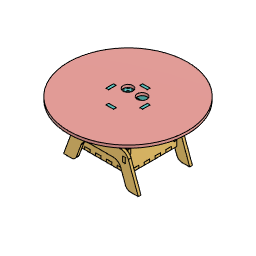
finalprojectbuild (Autodesk Fusion 360 design; units mm, degrees)
Autodesk Fusion 360 part; units mm, degrees
(part 1 of 2)
sketch "Sketch1" plane through (0, 0, 0) normal (1, 0, 0) x (0, 1, 0)
  line L0 (45, 50) -> (40, 50)
  line L1 (50, 45) -> (55, 45)
  line L2 (65, 50) -> (60, 50)
  line L3 (35, 45) -> (30, 45)
  line L4 (20, 50) -> (25, 50)
  line L5 (15, 45) -> (10, 45)
  line L6 (70, 45) -> (75, 45)
  line L7 (45, 50) -> (40, 50)
  line L8 (65, 50) -> (60, 50)
  line L9 (0, 50) -> (5, 50)
  line L10 (20, 50) -> (25, 50)
  line L11 (25, 50) -> (20, 50)
  line L12 (5, 50) -> (0, 50)
  line L13 (45, 0) -> (40, 0)
  line L14 (65, 0) -> (60, 0)
  line L15 (65, 0) -> (60, 0)
  line L16 (20, 0) -> (25, 0)
  line L17 (45, 0) -> (40, 0)
  line L18 (20, 0) -> (25, 0)
  line L19 (25, 0) -> (20, 0)
  line L20 (0, 0) -> (5, 0)
  line L21 (20, 0) -> (25, 0)
  line L22 (40, 0) -> (45, 0)
  line L23 (60, 0) -> (65, 0)
  line L24 (5, 30) -> (0, 30)
  line L25 (0, 20) -> (5, 20)
  line L26 (5, 20) -> (0, 20)
  line L27 (0, 10) -> (5, 10)
  line L28 (5, 10) -> (5, 20)
  line L29 (5, 30) -> (0, 30)
  line L30 (0, 40) -> (5, 40)
  line L31 (5, 40) -> (5, 30)
  line L32 (0, 20) -> (-5, 20)
  line L33 (-5, 20) -> (-5, 30)
  line L34 (-5, 30) -> (0, 30)
  line L35 (0, 50) -> (0, 40)
  line L36 (0, 10) -> (0, 0)
  line L37 (0, 50) -> (0, 40)
  line L38 (80, 45) -> (80, 50)
  line L39 (5, 50) -> (10, 50)
  line L40 (10, 50) -> (10, 45)
  line L41 (20, 50) -> (20, 45)
  line L42 (20, 45) -> (10, 45)
  line L43 (10, 45) -> (10, 50)
  line L44 (30, 45) -> (30, 50)
  line L45 (30, 50) -> (20, 50)
  line L46 (20, 50) -> (20, 45)
  line L47 (40, 50) -> (40, 45)
  line L48 (40, 45) -> (30, 45)
  line L49 (30, 45) -> (30, 50)
  line L50 (50, 45) -> (50, 50)
  line L51 (50, 50) -> (40, 50)
  line L52 (40, 50) -> (40, 45)
  line L53 (50, 45) -> (60, 45)
  line L54 (60, 45) -> (60, 50)
  line L55 (50, 50) -> (50, 45)
  line L56 (70, 45) -> (70, 50)
  line L57 (70, 50) -> (60, 50)
  line L58 (60, 50) -> (60, 45)
  line L59 (70, 45) -> (80, 45)
  line L60 (80, 45) -> (80, 50)
  line L61 (70, 50) -> (70, 45)
  line L62 (90, 45) -> (90, 50)
  line L63 (90, 50) -> (80, 50)
  line L64 (80, 50) -> (80, 45)
  line L65 (80, 45) -> (75, 45)
  line L66 (80, 0) -> (90, 0)
  line L67 (85, 40) -> (85, 30)
  line L68 (90, 10) -> (85, 10)
  line L69 (85, 30) -> (90, 30)
  line L70 (85, 30) -> (90, 30)
  line L71 (85, 20) -> (90, 20)
  line L72 (95, 20) -> (95, 30)
  line L73 (95, 30) -> (90, 30)
  line L74 (85, 10) -> (85, 20)
  line L75 (90, 20) -> (95, 20)
  line L76 (90, 40) -> (85, 40)
  line L77 (90, 20) -> (85, 20)
  line L78 (90, 40) -> (90, 45)
  line L79 (90, 0) -> (90, 10)
  line L80 (90, 50) -> (90, 25)
  line L81 (90, 25) -> (58, 25)
  line L82 (40, 5) -> (30, 5)
  line L83 (20, 0) -> (25, 0)
  line L84 (40, 0) -> (40, 5)
  line L85 (30, 5) -> (30, 0)
  line L86 (50, 5) -> (55, 5)
  line L87 (70, 5) -> (75, 5)
  line L88 (35, 5) -> (30, 5)
  line L89 (15, 5) -> (10, 5)
  line L90 (70, 0) -> (60, 0)
  line L91 (45, 0) -> (40, 0)
  line L92 (30, 0) -> (20, 0)
  line L93 (10, 0) -> (10, 5)
  line L94 (80, 5) -> (80, 0)
  line L95 (50, 5) -> (60, 5)
  line L96 (40, 0) -> (40, 5)
  line L97 (65, 0) -> (60, 0)
  line L98 (10, 5) -> (10, 0)
  line L99 (50, 0) -> (40, 0)
  line L100 (70, 0) -> (70, 5)
  line L101 (80, 5) -> (75, 5)
  line L102 (70, 5) -> (80, 5)
  line L103 (20, 0) -> (25, 0)
  line L104 (45, 0) -> (40, 0)
  line L105 (80, 5) -> (80, 0)
  line L106 (20, 0) -> (20, 5)
  line L107 (70, 5) -> (70, 0)
  line L108 (60, 0) -> (60, 5)
  line L109 (65, 0) -> (60, 0)
  line L110 (80, 0) -> (80, 5)
  line L111 (20, 0) -> (20, 5)
  line L112 (20, 5) -> (10, 5)
  line L113 (50, 0) -> (50, 5)
  line L114 (30, 5) -> (30, 0)
  line L115 (25, 0) -> (20, 0)
  line L116 (60, 5) -> (60, 0)
  line L117 (50, 5) -> (50, 0)
  line L118 (5, 0) -> (10, 0)
  line L119 (20, 0) -> (30, 0)
  line L120 (40, 0) -> (50, 0)
  line L121 (60, 0) -> (70, 0)
  line L122 (80, 0) -> (90, 0)
  dimension "d1" = 80
  dimension "d2" = 50
  dimension "d3" = 40
  dimension "d19" = 5
  dimension "d20" = 10
  dimension "d21" = 5
  dimension "d22" = 10
  dimension "d23" = 5
  dimension "d24" = 10
  dimension "d55" = 5
  dimension "d57" = 10
  dimension "d58" = 5
  dimension "d59" = 10
  dimension "d60" = 5
  dimension "d61" = 10
  dimension "d62" = 5
  dimension "d63" = 10
  dimension "d64" = 10
  dimension "d65" = 10
  dimension "d66" = 10
  dimension "d67" = 10
  dimension "d73" = 85
  dimension "d74" = 25
  dimension "d75" = 32
  constraint horizontal L20
  constraint vertical L35
  constraint coincident L20.start L36.end
  constraint perpendicular L9 L35
  constraint horizontal L0
  constraint horizontal L1
  constraint horizontal L2
  constraint horizontal L3
  constraint horizontal L4
  constraint horizontal L5
  constraint horizontal L6
  constraint collinear L9 L10
  constraint collinear L11 L12
  constraint perpendicular L5 L37
  constraint collinear L20 L21
  constraint collinear L21 L22
  constraint collinear L22 L23
  constraint horizontal L24
  constraint horizontal L25
  constraint horizontal L26
  constraint horizontal L27
  constraint vertical L28
  constraint horizontal L29
  constraint horizontal L30
  constraint vertical L31
  constraint horizontal L32
  constraint vertical L33
  constraint horizontal L34
  constraint collinear L35 L36
  constraint horizontal L39
  constraint vertical L40
  constraint vertical L41
  constraint horizontal L42
  constraint vertical L43
  constraint vertical L44
  constraint horizontal L45
  constraint vertical L46
  constraint vertical L47
  constraint horizontal L48
  constraint vertical L49
  constraint vertical L50
  constraint horizontal L51
  constraint vertical L52
  constraint horizontal L53
  constraint vertical L54
  constraint vertical L55
  constraint vertical L56
  constraint horizontal L57
  constraint vertical L58
  constraint horizontal L59
  constraint vertical L60
  constraint vertical L61
  constraint vertical L62
  constraint horizontal L63
  constraint vertical L64
  constraint horizontal L65
  constraint horizontal L66
  constraint vertical L79
  constraint collinear L78 L79
  constraint perpendicular L79 L118
  constraint perpendicular L73 L80
  constraint perpendicular L80 L81
  constraint symmetric L38.end L81 L66.start
  constraint symmetric L0.end L81 L13.end
  constraint symmetric L3.start L81 L88.start
  constraint symmetric L0.start L81 L13.start
  constraint symmetric L1.end L81 L86.end
  constraint symmetric L2.start L81 L14.start
  constraint symmetric L4.end L81 L16.end
  constraint symmetric L5.start L81 L89.start
  constraint symmetric L6.end L81 L87.end
  constraint symmetric L39.end L81 L93.start
  constraint symmetric L5.end L81 L89.end
  constraint symmetric L4.start L81 L16.start
  constraint symmetric L41.end L81 L106.end
  constraint symmetric L3.end L81 L82.end
  constraint symmetric L44.end L81 L85.end
  constraint symmetric L47.end L81 L82.start
  constraint symmetric L1.start L81 L86.start
  constraint symmetric L50.end L81 L99.start
  constraint symmetric L53.end L81 L95.end
  constraint symmetric L2.end L81 L14.end
  constraint symmetric L6.start L81 L87.start
  constraint symmetric L56.end L81 L90.start
  constraint symmetric L38.start L81 L94.start
  constraint collinear L118 L119
  constraint collinear L119 L120
  constraint collinear L120 L121
  constraint collinear L121 L122
  measures "d1" distance of L20.start L66.start
  measures "d2" distance of L20.start L9.start
  measures "d3" distance of L9.start L0.end
  measures "d19" distance of L25.end L25.start
  measures "d20" distance of L25.end L27.end
  measures "d21" distance of L24.start L24.end
  measures "d22" distance of L24.start L30.end
  measures "d23" distance of L25.start L32.end
  measures "d24" distance of L25.start L24.end
  measures "d55" distance of L9.end L39.end
  measures "d57" distance of L39.end L4.start
  measures "d58" distance of L39.end L5.end
  measures "d59" distance of L41.end L3.end
  measures "d60" distance of L41.end L4.start
  measures "d61" distance of L44.end L0.end
  measures "d62" distance of L44.end L3.end
  measures "d63" distance of L47.end L1.start
  measures "d64" distance of L1.start L53.end
  measures "d65" distance of L53.end L6.start
  measures "d66" distance of L6.start L38.start
  measures "d67" distance of L38.start L62.start
  measures "d73" distance of L20.end L66.end
  measures "d74" distance of L62.end L80.end
  measures "d75" distance of L80.end L81.end
extrude "Extrude1" add sketch "Sketch1" along normal blind 5 contours L0 L1 L2 L3 L4 L5 L6 L7 L8 L9 L10 L11 L12 L13 L14 L15 L16 L17 L18 L19 L20 L21 L22 L23 L24 L25 L26 L27 L28 L29 L30 L31 L32 L33 L34 L35 L36 L37 L38 L39 L40 L41 L42 L43 L44 L45 L46 L47 L48 L49 L50 L51 L52 L53 L54 L55 L56 L57 L58 L59 L60 L61 L62 L63 L64 L65 L66 L67 L68 L69 L70 L71 L72 L73 L74 L75 L76 L77 L78 L79 L80 L82 L83 L84 L85 L86 L87 L88 L89 L90 L91 L92 L93 L94 L95 L96 L97 L98 L99 L100 L101 L102 L103 L104 L105 L106 L107 L108 L109 L110 L111 L112 L113 L114 L115 L116 L117 L118 L119 L120 L121 L122 makes body 1
ref_plane "WorkPlane1" through (45, 45, 25) normal (1, 0, 0) x (0, 0, -1)
mirror "Mirror1" about plane through (45, 45, 25) normal (1, 0, 0) of bodies 1 makes body 2
sketch "Sketch2" plane through (0, 0, 0) normal (0, 1, 0) x (1, 0, 0)
  line L0 (90, -30) -> (85, -30)
  line L1 (85, -30) -> (85, -25)
  line L2 (90, -30) -> (85, -30)
  line L3 (85, -40) -> (90, -40)
  line L4 (90, -40) -> (90, -30)
  line L5 (90, -20) -> (85, -20)
  line L6 (85, -20) -> (85, -25)
  line L7 (90, -20) -> (85, -20)
  line L8 (85, -10) -> (90, -10)
  line L9 (90, -10) -> (90, -20)
  line L10 (85, -40) -> (85, -50)
  line L11 (85, -50) -> (85, -40)
  line L12 (85, -30) -> (85, -25)
  line L13 (85, 0) -> (85, -10)
  line L14 (85, -20) -> (85, -30)
  line L15 (0, -20) -> (5, -20)
  line L16 (5, -30) -> (5, -25)
  line L17 (5, -30) -> (5, -25)
  line L18 (0, -10) -> (0, -20)
  line L19 (5, -20) -> (5, -30)
  line L20 (5, -20) -> (5, -25)
  line L21 (0, -20) -> (5, -20)
  line L22 (0, -30) -> (5, -30)
  line L23 (0, -40) -> (0, -30)
  line L24 (5, -40) -> (0, -40)
  line L25 (0, -30) -> (5, -30)
  line L26 (5, -10) -> (0, -10)
  line L27 (5, -50) -> (5, -40)
  line L28 (5, -30) -> (5, -20)
  line L29 (5, -10) -> (5, 0)
  line L30 (45, -50) -> (50, -50)
  line L31 (50, -50) -> (50, -45)
  line L32 (45, -50) -> (40, -50)
  line L33 (40, -50) -> (40, -45)
  line L34 (50, -45) -> (60, -45)
  line L35 (60, -45) -> (60, -50)
  line L36 (50, -50) -> (50, -45)
  line L37 (70, -45) -> (70, -50)
  line L38 (70, -50) -> (60, -50)
  line L39 (60, -50) -> (60, -45)
  line L40 (70, -45) -> (80, -45)
  line L41 (80, -45) -> (80, -50)
  line L42 (70, -50) -> (70, -45)
  line L43 (40, -45) -> (30, -45)
  line L44 (30, -45) -> (30, -50)
  line L45 (40, -50) -> (40, -45)
  line L46 (20, -45) -> (20, -50)
  line L47 (20, -50) -> (30, -50)
  line L48 (30, -50) -> (30, -45)
  line L49 (20, -45) -> (10, -45)
  line L50 (10, -45) -> (10, -50)
  line L51 (20, -50) -> (20, -45)
  line L52 (10, -50) -> (5, -50)
  line L53 (30, -50) -> (20, -50)
  line L54 (50, -50) -> (45, -50)
  line L55 (50, -50) -> (40, -50)
  line L56 (85, -50) -> (80, -50)
  line L57 (70, -50) -> (60, -50)
  line L58 (85, -50) -> (80, -50)
  line L59 (70, -50) -> (60, -50)
  line L60 (70, 0) -> (60, 0)
  line L61 (20, 0) -> (20, -5)
  line L62 (20, 0) -> (30, 0)
  line L63 (60, -5) -> (60, 0)
  line L64 (30, -5) -> (30, 0)
  line L65 (70, 0) -> (60, 0)
  line L66 (20, -5) -> (10, -5)
  line L67 (60, 0) -> (60, -5)
  line L68 (40, -5) -> (30, -5)
  line L69 (50, -5) -> (60, -5)
  line L70 (40, 0) -> (40, -5)
  line L71 (45, 0) -> (40, 0)
  line L72 (30, 0) -> (20, 0)
  line L73 (30, 0) -> (30, -5)
  line L74 (45, 0) -> (50, 0)
  line L75 (20, -5) -> (20, 0)
  line L76 (70, -5) -> (80, -5)
  line L77 (40, 0) -> (40, -5)
  line L78 (50, 0) -> (40, 0)
  line L79 (70, 0) -> (60, 0)
  line L80 (10, -5) -> (10, 0)
  line L81 (70, -5) -> (70, 0)
  line L82 (80, -5) -> (80, 0)
  line L83 (50, 0) -> (45, 0)
  line L84 (70, 0) -> (70, -5)
  line L85 (50, 0) -> (50, -5)
  line L86 (50, 0) -> (50, -5)
  line L87 (5, 0) -> (10, 0)
  line L88 (20, 0) -> (30, 0)
  line L89 (40, 0) -> (50, 0)
  line L90 (60, 0) -> (70, 0)
  line L91 (80, 0) -> (85, 0)
  dimension "d31" = 80
  dimension "d32" = 50
  dimension "d33" = 25
  dimension "d34" = 40
  dimension "d36" = 5
  dimension "d37" = 10
  dimension "d39" = 5
  dimension "d40" = 10
  dimension "d41" = 5
  dimension "d43" = 5
  dimension "d45" = 10
  dimension "d46" = 10
  dimension "d47" = 10
  dimension "d48" = 10
  dimension "d49" = 10
  dimension "d50" = 10
  constraint horizontal L87
  constraint vertical L13
  constraint horizontal L58
  constraint vertical L27
  constraint perpendicular L11 L58
  constraint perpendicular L13 L56
  constraint horizontal L0
  constraint vertical L1
  constraint horizontal L2
  constraint horizontal L3
  constraint vertical L4
  constraint horizontal L5
  constraint vertical L6
  constraint horizontal L7
  constraint horizontal L8
  constraint vertical L9
  constraint collinear L10 L13
  constraint collinear L11 L12
  constraint collinear L13 L14
  constraint collinear L27 L28
  constraint collinear L28 L29
  constraint horizontal L30
  constraint vertical L31
  constraint horizontal L32
  constraint vertical L33
  constraint horizontal L34
  constraint vertical L35
  constraint vertical L36
  constraint vertical L37
  constraint horizontal L38
  constraint vertical L39
  constraint horizontal L40
  constraint vertical L41
  constraint vertical L42
  constraint horizontal L43
  constraint vertical L44
  constraint vertical L45
  constraint vertical L46
  constraint horizontal L47
  constraint vertical L48
  constraint horizontal L49
  constraint vertical L50
  constraint vertical L51
  constraint collinear L52 L58
  constraint collinear L53 L58
  constraint collinear L54 L56
  constraint collinear L55 L58
  constraint collinear L56 L57
  constraint collinear L58 L59
  constraint collinear L87 L88
  constraint collinear L88 L89
  constraint collinear L89 L90
  constraint collinear L90 L91
  measures "d31" distance of L29.end L13.start
  measures "d32" distance of L29.end L27.start
  measures "d33" distance of L10.end L1.end
  measures "d34" distance of L10.end L30.start
  measures "d36" distance of L1.end L0.end
  measures "d37" distance of L0.start L3.end
  measures "d39" distance of L1.end L5.end
  measures "d40" distance of L5.start L8.end
  measures "d41" distance of L30.start L30.end
  measures "d43" distance of L30.start L32.end
  measures "d45" distance of L31.end L34.end
  measures "d46" distance of L34.end L37.start
  measures "d47" distance of L37.start L40.end
  measures "d48" distance of L33.end L43.end
  measures "d49" distance of L43.end L46.start
  measures "d50" distance of L46.start L49.end
extrude "Extrude2" add sketch "Sketch2" along normal blind 5 separate body makes body 3
ref_plane "WorkPlane2" through (45, 45, 25) normal (0, 1, 0) x (0, 0, 1)
mirror "Mirror2" about plane through (45, 45, 25) normal (0, 1, 0) of bodies 3 makes body 4
sketch "Sketch3" plane through (0, 0, 0) normal (0, 0, 1) x (1, 0, 0)
  line L0 (45, 85) -> (40, 85)
  line L1 (40, 85) -> (40, 90)
  line L2 (50, 90) -> (50, 85)
  line L3 (50, 85) -> (40, 85)
  line L4 (40, 85) -> (40, 90)
  line L5 (50, 90) -> (60, 90)
  line L6 (60, 90) -> (60, 85)
  line L7 (50, 85) -> (50, 90)
  line L8 (70, 90) -> (70, 85)
  line L9 (70, 85) -> (60, 85)
  line L10 (60, 85) -> (60, 90)
  line L11 (70, 90) -> (80, 90)
  line L12 (80, 90) -> (80, 85)
  line L13 (70, 85) -> (70, 90)
  line L14 (40, 90) -> (30, 90)
  line L15 (30, 90) -> (30, 85)
  line L16 (40, 85) -> (40, 90)
  line L17 (20, 90) -> (20, 85)
  line L18 (20, 85) -> (30, 85)
  line L19 (30, 85) -> (30, 90)
  line L20 (20, 90) -> (10, 90)
  line L21 (10, 90) -> (10, 85)
  line L22 (20, 85) -> (20, 90)
  line L23 (5, 85) -> (10, 85)
  line L24 (5, 85) -> (10, 85)
  line L25 (20, 85) -> (30, 85)
  line L26 (40, 85) -> (45, 85)
  line L27 (20, 85) -> (30, 85)
  line L28 (40, 85) -> (50, 85)
  line L29 (60, 85) -> (70, 85)
  line L30 (80, 85) -> (85, 85)
  line L31 (0, 40) -> (0, 30)
  line L32 (0, 50) -> (0, 60)
  line L33 (0, 70) -> (5, 70)
  line L34 (0, 20) -> (5, 20)
  line L35 (0, 30) -> (5, 30)
  line L36 (5, 20) -> (5, 30)
  line L37 (5, 60) -> (5, 70)
  line L38 (5, 20) -> (5, 30)
  line L39 (5, 40) -> (5, 50)
  line L40 (5, 40) -> (0, 40)
  line L41 (5, 50) -> (5, 40)
  line L42 (5, 20) -> (0, 20)
  line L43 (5, 45) -> (5, 40)
  line L44 (5, 40) -> (5, 45)
  line L45 (5, 70) -> (5, 60)
  line L46 (5, 30) -> (0, 30)
  line L47 (0, 70) -> (0, 80)
  line L48 (5, 40) -> (0, 40)
  line L49 (5, 60) -> (0, 60)
  line L50 (0, 10) -> (5, 10)
  line L51 (5, 40) -> (0, 40)
  line L52 (0, 50) -> (5, 50)
  line L53 (0, 20) -> (0, 10)
  line L54 (0, 60) -> (5, 60)
  line L55 (5, 50) -> (0, 50)
  line L56 (5, 70) -> (0, 70)
  line L57 (0, 80) -> (5, 80)
  line L58 (5, 20) -> (5, 30)
  line L59 (50, 0) -> (60, 0)
  line L60 (40, 0) -> (30, 0)
  line L61 (20, 0) -> (20, 5)
  line L62 (70, 0) -> (70, 5)
  line L63 (60, 0) -> (60, 5)
  line L64 (70, 5) -> (60, 5)
  line L65 (30, 5) -> (20, 5)
  line L66 (70, 5) -> (60, 5)
  line L67 (50, 5) -> (40, 5)
  line L68 (50, 5) -> (50, 0)
  line L69 (40, 5) -> (50, 5)
  line L70 (70, 5) -> (70, 0)
  line L71 (45, 5) -> (50, 5)
  line L72 (50, 5) -> (45, 5)
  line L73 (20, 5) -> (30, 5)
  line L74 (60, 5) -> (60, 0)
  line L75 (20, 0) -> (10, 0)
  line L76 (50, 5) -> (50, 0)
  line L77 (30, 5) -> (30, 0)
  line L78 (80, 0) -> (80, 5)
  line L79 (50, 5) -> (50, 0)
  line L80 (40, 0) -> (40, 5)
  line L81 (70, 0) -> (80, 0)
  line L82 (30, 0) -> (30, 5)
  line L83 (40, 5) -> (40, 0)
  line L84 (20, 5) -> (20, 0)
  line L85 (10, 0) -> (10, 5)
  line L86 (70, 5) -> (60, 5)
  line L87 (5, 80) -> (5, 85)
  line L88 (5, 80) -> (5, 85)
  line L89 (5, 60) -> (5, 70)
  line L90 (5, 45) -> (5, 50)
  line L91 (5, 60) -> (5, 70)
  line L92 (5, 40) -> (5, 50)
  line L93 (5, 5) -> (5, 10)
  line L94 (5, 20) -> (5, 30)
  line L95 (90, 30) -> (85, 30)
  line L96 (90, 20) -> (90, 10)
  line L97 (85, 40) -> (90, 40)
  line L98 (85, 20) -> (85, 30)
  line L99 (90, 40) -> (90, 30)
  line L100 (85, 60) -> (85, 70)
  line L101 (85, 20) -> (85, 30)
  line L102 (85, 30) -> (90, 30)
  line L103 (85, 50) -> (90, 50)
  line L104 (90, 70) -> (85, 70)
  line L105 (85, 40) -> (90, 40)
  line L106 (85, 70) -> (85, 60)
  line L107 (85, 50) -> (85, 40)
  line L108 (90, 50) -> (85, 50)
  line L109 (85, 40) -> (90, 40)
  line L110 (85, 45) -> (85, 40)
  line L111 (90, 20) -> (85, 20)
  line L112 (85, 40) -> (85, 50)
  line L113 (85, 20) -> (85, 30)
  line L114 (90, 70) -> (90, 80)
  line L115 (85, 60) -> (85, 70)
  line L116 (85, 20) -> (85, 30)
  line L117 (85, 20) -> (90, 20)
  line L118 (90, 10) -> (85, 10)
  line L119 (90, 60) -> (85, 60)
  line L120 (85, 40) -> (85, 50)
  line L121 (85, 60) -> (85, 70)
  line L122 (90, 50) -> (90, 60)
  line L123 (85, 60) -> (90, 60)
  line L124 (90, 80) -> (85, 80)
  line L125 (85, 40) -> (85, 45)
  line L126 (85, 70) -> (90, 70)
  line L127 (85, 45) -> (85, 50)
  line L128 (85, 85) -> (85, 80)
  line L129 (85, 70) -> (85, 60)
  line L130 (85, 50) -> (85, 40)
  line L131 (85, 30) -> (85, 20)
  line L132 (85, 10) -> (85, 5)
  line L133 (85, 5) -> (80, 5)
  line L134 (70, 5) -> (60, 5)
  line L135 (50, 5) -> (40, 5)
  line L136 (30, 5) -> (20, 5)
  line L137 (10, 5) -> (5, 5)
  dimension "d76" = 80
  dimension "d77" = 80
  dimension "d78" = 40
  dimension "d79" = 40
  dimension "d80" = 5
  dimension "d82" = 10
  dimension "d83" = 10
  dimension "d84" = 10
  dimension "d85" = 10
  dimension "d86" = 10
  dimension "d87" = 10
  dimension "d88" = 10
  constraint horizontal L24
  constraint vertical L128
  constraint horizontal L133
  constraint vertical L93
  constraint horizontal L23
  constraint vertical L90
  constraint horizontal L0
  constraint vertical L1
  constraint vertical L2
  constraint horizontal L3
  constraint vertical L4
  constraint horizontal L5
  constraint vertical L6
  constraint vertical L7
  constraint vertical L8
  constraint horizontal L9
  constraint vertical L10
  constraint horizontal L11
  constraint vertical L12
  constraint vertical L13
  constraint horizontal L14
  constraint vertical L15
  constraint vertical L16
  constraint vertical L17
  constraint horizontal L18
  constraint vertical L19
  constraint horizontal L20
  constraint vertical L21
  constraint vertical L22
  constraint collinear L23 L25
  constraint collinear L24 L27
  constraint collinear L25 L26
  constraint collinear L27 L28
  constraint collinear L28 L29
  constraint collinear L29 L30
  constraint collinear L87 L93
  constraint collinear L88 L90
  constraint collinear L89 L93
  constraint collinear L90 L91
  constraint collinear L92 L93
  constraint collinear L93 L94
  constraint collinear L128 L129
  constraint collinear L129 L130
  constraint collinear L130 L131
  constraint collinear L131 L132
  constraint collinear L133 L134
  constraint collinear L134 L135
  constraint collinear L135 L136
  constraint collinear L136 L137
  measures "d76" distance of L23.start L30.end
  measures "d77" distance of L23.start L93.start
  measures "d78" distance of L23.start L0.start
  measures "d79" distance of L23.start L43.start
  measures "d80" distance of L0.start L0.end
  measures "d82" distance of L1.end L2.start
  measures "d83" distance of L2.start L5.end
  measures "d84" distance of L5.end L8.start
  measures "d85" distance of L8.start L11.end
  measures "d86" distance of L1.end L14.end
  measures "d87" distance of L14.end L17.start
  measures "d88" distance of L17.start L20.end
extrude "Extrude3" add sketch "Sketch3" along normal blind 5 separate body makes body 5
ref_plane "WorkPlane3" through (45, 45, 25) normal (0, 0, 1) x (1, 0, 0)
mirror "Mirror3" about plane through (45, 45, 25) normal (0, 0, 1) of bodies 5 makes body 6
sketch "Sketch4" plane through (0, 0, 0) normal (0, -1, 0) x (1, 0, 0)
  line L0 (60, 5) -> (60, 0)
  line L1 (60, 0) -> (70, 0)
  line L2 (70, 0) -> (70, 5)
  line L3 (70, 5) -> (80, 5)
  line L4 (80, 5) -> (80, 0)
  line L5 (80, 0) -> (85, 0)
  line L6 (85, 0) -> (85, 10)
  line L7 (85, 10) -> (90, 10)
  line L8 (90, 20) -> (85, 20)
  line L9 (85, 20) -> (85, 30)
  line L10 (85, 30) -> (90, 30)
  line L11 (90, 40) -> (85, 40)
  line L12 (85, 40) -> (85, 50)
  line L13 (85, 50) -> (80, 50)
  line L14 (80, 50) -> (80, 45)
  line L15 (80, 45) -> (70, 45)
  line L16 (70, 45) -> (70, 50)
  line L17 (70, 50) -> (60, 50)
  line L18 (60, 50) -> (60, 45)
  line L19 (60, 45) -> (50, 45)
  line L20 (50, 45) -> (50, 50)
  line L21 (50, 50) -> (40, 50)
  line L22 (40, 50) -> (40, 45)
  line L23 (40, 45) -> (30, 45)
  line L24 (30, 45) -> (30, 50)
  line L25 (30, 50) -> (20, 50)
  line L26 (20, 50) -> (20, 45)
  line L27 (20, 45) -> (10, 45)
  line L28 (10, 45) -> (10, 50)
  line L29 (10, 50) -> (5, 50)
  line L30 (5, 50) -> (5, 40)
  line L31 (5, 40) -> (0, 40)
  line L32 (0, 30) -> (5, 30)
  line L33 (5, 30) -> (5, 20)
  line L34 (5, 20) -> (0, 20)
  line L35 (0, 10) -> (5, 10)
  line L36 (5, 10) -> (5, 0)
  line L37 (5, 0) -> (10, 0)
  line L38 (10, 0) -> (10, 5)
  line L39 (10, 5) -> (20, 5)
  line L40 (20, 5) -> (20, 0)
  line L41 (20, 0) -> (30, 0)
  line L42 (30, 0) -> (30, 5)
  line L43 (30, 5) -> (40, 5)
  line L44 (40, 5) -> (40, 0)
  line L45 (40, 0) -> (50, 0)
  line L46 (50, 0) -> (50, 5)
  line L47 (50, 5) -> (60, 5)
  line L48 (0, 0) -> (90, 0)
  line L49 (-2.0507, 39.3657) -> (-23.9414, -20.7785)
  line L50 (0, 45) -> (70, 45) construction
  line L51 (92.0507, 39.3657) -> (113.9414, -20.7785)
  line L52 (90, 45) -> (160, 45) construction
  line L53 (-2.0507, 39.3657) -> (-6.8404, 26.2061)
  line L54 (92.0507, 39.3657) -> (96.8404, 26.2061)
  line L55 (11.9534, 19.3657) -> (78.0466, 19.3657)
  line L56 (11.9534, 19.3657) -> (-2.6579, -20.7785)
  line L57 (78.0466, 19.3657) -> (92.6579, -20.7785)
  line L58 (-23.9414, -20.7785) -> (-2.6579, -20.7785)
  line L59 (92.6579, -20.7785) -> (113.9414, -20.7785)
  line L60 (0, 30) -> (5, 30)
  line L61 (5, 30) -> (5, 20)
  line L62 (5, 20) -> (0, 20)
  line L63 (0, 20) -> (0, 30)
  line L64 (90, 30) -> (85, 30)
  line L65 (85, 30) -> (85, 20)
  line L66 (85, 20) -> (90, 20)
  line L67 (90, 20) -> (90, 30)
  line L68 (27.0004, 39.3657) -> (-2.0507, 39.3657)
  line L69 (27.0004, 39.3657) -> (92.0507, 39.3657)
  dimension "d97" = 90
  dimension "d98" = 45
  dimension "d99" = 110
  dimension "d100" = 70
  dimension "d101" = 70
  dimension "d102" = 70
  dimension "d103" = 20
  dimension "d104" = 20
  dimension "d105" = 20
  dimension "d106" = 20
  dimension "d109" = 5
  dimension "d110" = 10
  dimension "d111" = 5
  dimension "d112" = 10
  constraint horizontal L48
  constraint coincident L48.start origin
  constraint horizontal L50
  constraint horizontal L52
  constraint parallel L49 L53
  constraint parallel L51 L54
  constraint collinear L58 L59
  constraint horizontal L60
  constraint vertical L61
  constraint horizontal L62
  constraint vertical L63
  constraint coincident L32.start L60.start
  constraint horizontal L64
  constraint vertical L65
  constraint horizontal L66
  constraint vertical L67
  constraint coincident L10.end L64.start
  measures "d97" distance of L48.start L48.end
  measures "d98" distance of L48.start L50.start
  measures "d99" angle of L49 L50
  measures "d100" distance of L50.start L49.end
  measures "d101" angle of L51 L52
  measures "d102" distance of L52.start L51.end
  measures "d103" distance of L50.start L53.end
  measures "d104" distance of L53.end L55.start
  measures "d105" distance of L52.start L54.end
  measures "d106" distance of L54.end L55.end
  measures "d109" distance of L32.start L32.end
  measures "d110" distance of L32.start L34.end
  measures "d111" distance of L10.end L9.end
  measures "d112" distance of L10.end L8.start
extrude "Extrude4" add sketch "Sketch4" along normal blind 5 separate body contours L49 L51 L53 L54 L55 L56 L57 L58 L59 L68 L69 makes body 7
fillet "Fillet1" radius 15 4 edges at (92.0507, -2.5, 39.3657) (-2.0507, -2.5, 39.3657) (11.9534, -2.5, 19.3657) (78.0466, -2.5, 19.3657) on bodies 7
fillet "Fillet2" radius 10 2 edges at (-2.6579, -2.5, -20.7785) (92.6579, -2.5, -20.7785) on bodies 7
mirror "Mirror4" about plane through (45, 45, 25) normal (0, 1, 0) of bodies 7 makes body 8
sketch "Sketch5" plane through (0, 0, 50) normal (0, 0, 1) x (-1, 0, 0)
  line L0 (-50, -5) -> (-50, 0)
  line L1 (-50, 0) -> (-60, 0)
  line L2 (-60, 0) -> (-60, -5)
  line L3 (-60, -5) -> (-70, -5)
  line L4 (-70, -5) -> (-70, 0)
  line L5 (-70, 0) -> (-80, 0)
  line L6 (-80, 0) -> (-80, -5)
  line L7 (-80, -5) -> (-85, -5)
  line L8 (-85, -5) -> (-85, -10)
  line L9 (-85, -10) -> (-90, -10)
  line L10 (-90, -10) -> (-90, -20)
  line L11 (-90, -20) -> (-85, -20)
  line L12 (-85, -20) -> (-85, -30)
  line L13 (-85, -30) -> (-90, -30)
  line L14 (-90, -30) -> (-90, -40)
  line L15 (-90, -40) -> (-85, -40)
  line L16 (-85, -40) -> (-85, -50)
  line L17 (-85, -50) -> (-90, -50)
  line L18 (-90, -50) -> (-90, -60)
  line L19 (-90, -60) -> (-85, -60)
  line L20 (-85, -60) -> (-85, -70)
  line L21 (-85, -70) -> (-90, -70)
  line L22 (-90, -70) -> (-90, -80)
  line L23 (-90, -80) -> (-85, -80)
  line L24 (-85, -80) -> (-85, -85)
  line L25 (-85, -85) -> (-80, -85)
  line L26 (-80, -85) -> (-80, -90)
  line L27 (-80, -90) -> (-70, -90)
  line L28 (-70, -90) -> (-70, -85)
  line L29 (-70, -85) -> (-60, -85)
  line L30 (-60, -85) -> (-60, -90)
  line L31 (-60, -90) -> (-50, -90)
  line L32 (-50, -90) -> (-50, -85)
  line L33 (-50, -85) -> (-40, -85)
  line L34 (-40, -85) -> (-40, -90)
  line L35 (-40, -90) -> (-30, -90)
  line L36 (-30, -90) -> (-30, -85)
  line L37 (-30, -85) -> (-20, -85)
  line L38 (-20, -85) -> (-20, -90)
  line L39 (-20, -90) -> (-10, -90)
  line L40 (-10, -90) -> (-10, -85)
  line L41 (-10, -85) -> (-5, -85)
  line L42 (-5, -85) -> (-5, -80)
  line L43 (-5, -80) -> (0, -80)
  line L44 (0, -80) -> (0, -70)
  line L45 (0, -70) -> (-5, -70)
  line L46 (-5, -70) -> (-5, -60)
  line L47 (-5, -60) -> (0, -60)
  line L48 (0, -60) -> (0, -50)
  line L49 (0, -50) -> (-5, -50)
  line L50 (-5, -50) -> (-5, -40)
  line L51 (-5, -40) -> (0, -40)
  line L52 (0, -40) -> (0, -30)
  line L53 (0, -30) -> (-5, -30)
  line L54 (-5, -30) -> (-5, -20)
  line L55 (-5, -20) -> (0, -20)
  line L56 (0, -20) -> (0, -10)
  line L57 (0, -10) -> (-5, -10)
  line L58 (-5, -10) -> (-5, -5)
  line L59 (-5, -5) -> (-10, -5)
  line L60 (-10, -5) -> (-10, 0)
  line L61 (-10, 0) -> (-20, 0)
  line L62 (-20, 0) -> (-20, -5)
  line L63 (-20, -5) -> (-30, -5)
  line L64 (-30, -5) -> (-30, 0)
  line L65 (-30, 0) -> (-40, 0)
  line L66 (-40, 0) -> (-40, -5)
  line L67 (-40, -5) -> (-50, -5)
  line L68 (0, -90) -> (-45, -90)
  line L69 (0, -45) -> (0, -90)
  line L70 (-6, -45) -> (-6, -84)
  line L71 (-6, -84) -> (-45, -84)
  line L72 (-6, -84) -> (-84, -84)
  line L73 (-84, -84) -> (-84, -6)
  line L74 (-84, -6) -> (-6, -6)
  line L75 (-6, -6) -> (-6, -84)
  dimension "d124" = 45
  dimension "d125" = 45
  dimension "d131" = 78
  dimension "d132" = 78
  constraint horizontal L68
  constraint vertical L69
  constraint vertical L70
  constraint horizontal L71
  constraint horizontal L72
  constraint vertical L73
  constraint horizontal L74
  constraint vertical L75
  measures "d124" distance of L68.start L68.end
  measures "d125" distance of L68.start L69.start
  measures "d131" distance of L70.end L72.end
  measures "d132" distance of L70.end L74.end
ref_plane "WorkPlane4" through (45, 45, 75) normal (0, 0, 1) x (-1, 0, 0)
sketch "Sketch6" plane through (45, 45, 75) normal (0, 0, 1) x (1, 0, 0)
  circle A0 centre (0, 0) radius 37.5
  dimension "d128" = 75
  constraint coincident A0.centre origin
  measures "d128" diameter of A0
loft "Loft1" add profiles "Sketch5", "Sketch6" section 1 contours L70 L71 L72 L73 L74 L75 section 2 separate body makes body 9 in component "Component"
sketch "Sketch7" plane through (0, 0, 75) normal (0, 0, 1) x (-1, 0, 0)
  arc A0 (-18.4835, -18.4835) -> (-71.5165, -18.4835) centre (-45, -45) ccw
  arc A1 (-71.5165, -18.4835) -> (-71.5165, -71.5165) centre (-45, -45) ccw
  arc A2 (-71.5165, -71.5165) -> (-18.4835, -71.5165) centre (-45, -45) ccw
  arc A3 (-18.4835, -71.5165) -> (-18.4835, -18.4835) centre (-45, -45) ccw
  line L0 (-20, -45) -> (-20, -70)
  line L1 (-20, -70) -> (-45, -70)
  line L2 (-20, -70) -> (-70, -70)
  line L3 (-70, -70) -> (-70, -20)
  line L4 (-70, -20) -> (-20, -20)
  line L5 (-20, -20) -> (-20, -70)
  dimension "d133" = 25
  dimension "d134" = 25
  dimension "d135" = 50
  dimension "d136" = 50
  constraint vertical L0
  constraint horizontal L1
  constraint horizontal L2
  constraint vertical L3
  constraint horizontal L4
  constraint vertical L5
  measures "d133" distance of A0.centre L0.start
  measures "d134" distance of A0.centre L1.end
  measures "d135" distance of L0.end L2.end
  measures "d136" distance of L0.end L4.end
extrude "Extrude1'" cut sketch "Sketch7" against normal blind 14 contours L0 L1 L2 L3 L4 L5 bodies 9 in component "Component"
sketch "Sketch8" plane through (0, 0, 75) normal (0, 0, 1) x (-1, 0, 0)
  line L0 (-70, -70) -> (-70, -20)
  line L1 (-70, -20) -> (-20, -20)
  line L2 (-20, -20) -> (-20, -70)
  line L3 (-20, -70) -> (-70, -70)
  arc A0 (-18.4835, -18.4835) -> (-71.5165, -18.4835) centre (-45, -45) ccw
  arc A1 (-71.5165, -18.4835) -> (-71.5165, -71.5165) centre (-45, -45) ccw
  arc A2 (-71.5165, -71.5165) -> (-18.4835, -71.5165) centre (-45, -45) ccw
  arc A3 (-18.4835, -71.5165) -> (-18.4835, -18.4835) centre (-45, -45) ccw
  circle A4 centre (-45, -45) radius 110
  dimension "d139" = 220
  constraint concentric A0 A4
  measures "d139" diameter of A4
extrude "Extrude1''" add sketch "Sketch8" along normal blind 5 separate body contours L0 L1 L2 L3 | A0 A1 A2 A3 | A4 makes body 10 in component "Component'"
sketch "Sketch9" plane through (0, 0, 75) normal (0, 0, 1) x (-1, 0, 0)
  line L0 (-70, -70) -> (-70, -20)
  line L1 (-70, -20) -> (-20, -20)
  line L2 (-20, -20) -> (-20, -70)
  line L3 (-20, -70) -> (-70, -70)
  arc A0 (-18.4835, -18.4835) -> (-71.5165, -18.4835) centre (-45, -45) ccw
  arc A1 (-71.5165, -18.4835) -> (-71.5165, -71.5165) centre (-45, -45) ccw
  arc A2 (-71.5165, -71.5165) -> (-18.4835, -71.5165) centre (-45, -45) ccw
  arc A3 (-18.4835, -71.5165) -> (-18.4835, -18.4835) centre (-45, -45) ccw
  line L4 (-20, -70) -> (-70, -70)
  line L5 (-70, -70) -> (-70, -20)
  line L6 (-70, -20) -> (-20, -20)
  line L7 (-20, -20) -> (-20, -70)
  line L8 (-62.5, -77.5) -> (-62.5, -62.5)
  line L9 (-62.5, -62.5) -> (-77.5, -62.5)
  line L10 (-62.5, -62.5) -> (-82.5, -62.5)
  line L11 (-82.5, -62.5) -> (-82.5, -82.5)
  line L12 (-82.5, -82.5) -> (-62.5, -82.5)
  line L13 (-62.5, -82.5) -> (-62.5, -62.5)
  dimension "d146" = 20
  dimension "d147" = 20
  constraint horizontal L4
  constraint vertical L5
  constraint horizontal L6
  constraint vertical L7
  constraint coincident L0.end L1.start
  constraint coincident L2.end L3.start
  constraint vertical L8
  constraint horizontal L9
  constraint horizontal L10
  constraint vertical L11
  constraint horizontal L12
  constraint vertical L13
  measures "d146" distance of L8.end L10.end
  measures "d147" distance of L8.end L12.end
extrude "Extrude2'" cut sketch "Sketch9" against normal blind 10 contours L0 L3 A1 A2 L4 L5 L8 L9 L10 L13 | L0 L3 L4 L5 L8 L9 L10 L13 | A1 A2 L10 L11 L12 L13 bodies 9 in component "Component"
pattern_circular "C-Pattern1" count 4 over 360 about axis through (45, 45, 75) along (0, 0, -1) of "Extrude2'" in component "Component"
sketch "Sketch10" plane through (0, 0, 75) normal (0, 0, 1) x (-1, 0, 0)
  line L0 (-27.5, -78.1662) -> (-27.5, -70)
  line L1 (-27.5, -70) -> (-62.5, -70)
  line L2 (-62.5, -70) -> (-62.5, -78.1662)
  arc A0 (-62.5, -78.1662) -> (-27.5, -78.1662) centre (-45, -45) ccw
  line L3 (-20, -70) -> (-45, -70)
  line L4 (-45, -70) -> (-45, -73.75)
  line L5 (-45, -73.75) -> (-38, -73.75)
  line L6 (-38, -73.75) -> (-38, -78.75)
  line L7 (-38, -78.75) -> (-45, -78.75)
  line L8 (-38, -73.75) -> (-52, -73.75)
  line L9 (-52, -73.75) -> (-52, -78.75)
  line L10 (-52, -78.75) -> (-38, -78.75)
  line L11 (-38, -78.75) -> (-38, -73.75)
  dimension "d152" = 25
  dimension "d153" = 3.75
  dimension "d154" = 7
  dimension "d155" = 5
  dimension "d156" = 14
  dimension "d157" = 5
  constraint perpendicular L0 L3
  constraint perpendicular L3 L4
  constraint horizontal L5
  constraint vertical L6
  constraint horizontal L7
  constraint horizontal L8
  constraint vertical L9
  constraint horizontal L10
  constraint vertical L11
  measures "d152" distance of L3.start L3.end
  measures "d153" distance of L3.end L4.end
  measures "d154" distance of L4.end L5.end
  measures "d155" distance of L4.end L7.end
  measures "d156" distance of L5.end L8.end
  measures "d157" distance of L5.end L6.end
extrude "Extrude3'" add sketch "Sketch10" along normal blind 5 contours L5 L6 L7 L8 L9 L10 L11 bodies 9 in component "Component"
pattern_circular "C-Pattern2" count 4 over 360 about axis through (45, 45, 75) along (0, 0, -1) of "Extrude3'" in component "Component"
sketch "Sketch11" plane through (0, 0, 80) normal (0, 0, 1) x (-1, 0, 0)
  circle A0 centre (-45, -45) radius 110
  circle A1 centre (-45, -45) radius 37.5
  line L0 (-82.5, -45) -> (-82.5, -7.5)
  line L1 (-82.5, -7.5) -> (-45, -7.5)
  line L2 (-45, -7.5) -> (-45, -45)
  line L3 (-82.5, -45) -> (-78.75, -45)
  line L4 (-73.75, -45) -> (-73.75, -52)
  line L5 (-73.75, -52) -> (-78.75, -52)
  line L6 (-78.75, -52) -> (-78.75, -45)
  line L7 (-73.75, -52) -> (-78.75, -52)
  line L8 (-78.75, -52) -> (-78.75, -38)
  line L9 (-78.75, -38) -> (-73.75, -38)
  line L10 (-73.75, -38) -> (-73.75, -52)
  line L11 (-45, -45) -> (-73.75, -45)
  line L12 (-78.75, -45) -> (-82.5, -45)
  dimension "d162" = 75
  dimension "d163" = 37.5
  dimension "d164" = 37.5
  dimension "d165" = 3.75
  dimension "d166" = 5
  dimension "d167" = 5
  dimension "d168" = 14
  constraint concentric A0 A1
  constraint horizontal L11
  constraint vertical L0
  constraint horizontal L1
  constraint vertical L2
  constraint coincident A0.centre A1.centre
  constraint perpendicular L0 L3
  constraint vertical L4
  constraint horizontal L5
  constraint vertical L6
  constraint horizontal L7
  constraint vertical L8
  constraint horizontal L9
  constraint vertical L10
  constraint collinear L11 L12
  measures "d162" diameter of A1
  measures "d163" distance of A0.centre L0.start
  measures "d164" distance of A0.centre L1.end
  measures "d165" distance of L0.start L3.end
  measures "d166" distance of L3.end L4.start
  measures "d167" distance of L4.end L5.end
  measures "d168" distance of L4.end L9.end
extrude "Extrude2''" cut sketch "Sketch11" against normal blind 5 contours L4 L5 L6 L7 L8 L9 L10 bodies 10 in component "Component'"
pattern_circular "C-Pattern1'" count 4 over 360 about axis through (45, 45, 80) along (0, 0, 1) of "Extrude2''" in component "Component'"
sketch "Sketch12" plane through (0, 0, 75) normal (0, 0, 1) x (-1, 0, 0)
  line L0 (-78.75, -52) -> (-78.75, -38)
  line L1 (-78.75, -38) -> (-73.75, -38)
  line L2 (-73.75, -38) -> (-73.75, -52)
  line L3 (-73.75, -52) -> (-78.75, -52)
  line L4 (-70, -27.5) -> (-78.1662, -27.5)
  arc A0 (-78.1662, -27.5) -> (-78.1662, -62.5) centre (-45, -45) ccw
  line L5 (-78.1662, -62.5) -> (-70, -62.5)
  line L6 (-70, -62.5) -> (-70, -27.5)
  line L7 (-45, -45) -> (-20, -45)
  line L8 (-20, -45) -> (-20, -70)
  line L9 (-20, -70) -> (-45, -70)
  line L10 (-45, -70) -> (-45, -45)
  line L11 (-45, -70) -> (-45, -67)
  line L12 (-45, -67) -> (-20, -67)
  line L13 (-20, -67) -> (-20, -49)
  line L14 (-20, -49) -> (-45, -49)
  line L15 (-45, -49) -> (-45, -67)
  line L16 (-45, -67) -> (-41, -67)
  line L17 (-41, -67) -> (-41, -58)
  line L18 (-41, -58) -> (-45, -58)
  line L19 (-45, -58) -> (-45, -67)
  circle A1 centre (-32, -58) radius 9
  circle A2 centre (-58, -58) radius 9
  dimension "d173" = 25
  dimension "d174" = 25
  dimension "d175" = 3
  dimension "d176" = 25
  dimension "d177" = 18
  dimension "d178" = 4
  dimension "d179" = 9
  dimension "d180" = 9
  dimension "d181" = 18
  constraint horizontal L7
  constraint vertical L8
  constraint horizontal L9
  constraint vertical L10
  constraint coincident A0.centre L7.start
  constraint perpendicular L9 L11
  constraint horizontal L12
  constraint vertical L13
  constraint horizontal L14
  constraint vertical L15
  constraint horizontal L16
  constraint vertical L17
  constraint horizontal L18
  constraint vertical L19
  constraint symmetric L10 A1 A2
  measures "d173" distance of A0.centre L7.end
  measures "d174" distance of A0.centre L9.end
  measures "d175" distance of L9.end L11.end
  measures "d176" distance of L11.end L12.end
  measures "d177" distance of L11.end L14.end
  measures "d178" distance of L11.end L16.end
  measures "d179" distance of L11.end L18.end
  measures "d180" distance of L17.end A1.centre
  measures "d181" diameter of A1
extrude "Extrude3''" cut sketch "Sketch12" along normal blind 5 contours A1 | A2 bodies 10 in component "Component'"
sketch "Sketch13" plane through (0, 0, 61) normal (0, 0, 1) x (-1, 0, 0)
  line L0 (-20, -20) -> (-70, -20)
  line L1 (-70, -20) -> (-70, -70)
  line L2 (-70, -70) -> (-20, -70)
  line L3 (-20, -70) -> (-20, -20)
  line L4 (-20, -70) -> (-45, -70)
  line L5 (-20, -45) -> (-20, -70)
  circle A0 centre (-45, -45) radius 17.5
  dimension "d184" = 25
  dimension "d185" = 25
  dimension "d187" = 35
  constraint horizontal L4
  constraint vertical L5
  constraint coincident L2.end L3.start
  measures "d184" distance of L2.end L4.end
  measures "d185" distance of L2.end L5.start
  measures "d187" diameter of A0
extrude "Extrude5" cut sketch "Sketch13" against normal blind 50 contours A0 bodies 6
extrude "Extrude4'" cut sketch "Sketch13" against normal blind 50 contours A0 bodies 9 in component "Component"
sketch "Sketch14" plane through (0, 0, 65) normal (0, 0, 1) x (-1, 0, 0)
  spline S0 degree 3 poles (-13.4901, -13.4901) (-11.4888, -17.99) (-9.9418, -22.6941) (-8.8517, -27.5) knots -1.529594 -1.529594 -1.529594 -1.529594 -0.051231 -0.051231 -0.051231 -0.051231
  spline S1 degree 3 poles (-27.5, -8.8517) (-22.6941, -9.9418) (-17.99, -11.4888) (-13.4901, -13.4901) knots -1.477466 -1.477466 -1.477466 -1.477466 0 0 0 0
  line L0 (-27.5, -8.8517) -> (-27.5, -20)
  line L1 (-27.5, -20) -> (-20, -20)
  line L2 (-20, -20) -> (-20, -27.5)
  line L3 (-20, -27.5) -> (-8.8517, -27.5)
  circle A0 centre (-13.4901, -13.4901) radius 3
  dimension "d192" = 6
  constraint coincident S0.start S1.end
  measures "d192" diameter of A0
extrude "Extrude6" cut sketch "Sketch14" against normal blind 40 contours S0 S1 A0 | S0 S1 A0 bodies 6
extrude "Extrude5'" cut sketch "Sketch14" against normal blind 40 contours S0 S1 A0 | S0 S1 A0 bodies 9 in component "Component"
pattern_circular "C-Pattern1''" count 4 over 360 about axis through (45, 45, 75) along (0, 0, -1) of "Extrude6"
pattern_circular "C-Pattern3" count 4 over 360 about axis through (45, 45, 75) along (0, 0, -1) of "Extrude5'" in component "Component"
sketch "Sketch15" plane through (0, 0, 65) normal (0, 0, 1) x (-1, 0, 0)
  arc A0 (-12.3272, -73.7444) -> (-16.2556, -77.6728) centre (-13.4901, -76.5099) ccw
  spline S0 degree 3 poles (-8.8517, -62.5) (-9.7204, -66.3301) (-10.8794, -70.0955) (-12.3272, -73.7444) knots -1.477466 -1.477466 -1.477466 -1.477466 -0.299993 -0.299993 -0.299993 -0.299993
  line L0 (-8.8517, -62.5) -> (-20, -62.5)
  line L1 (-20, -62.5) -> (-20, -70)
  line L2 (-20, -70) -> (-27.5, -70)
  line L3 (-27.5, -70) -> (-27.5, -81.1483)
  spline S1 degree 3 poles (-16.2556, -77.6728) (-19.9045, -79.1206) (-23.6699, -80.2796) (-27.5, -81.1483) knots -1.229419 -1.229419 -1.229419 -1.229419 -0.051231 -0.051231 -0.051231 -0.051231
  line L4 (-18.4901, -76.5099) -> (-18.4901, -76.5089)
  line L5 (-13.4911, -71.5099) -> (-13.4901, -71.5099)
  line L6 (-13.4911, -71.5099) -> (1.5099, -71.5099)
  line L7 (1.5099, -71.5099) -> (1.5099, -91.5099)
  line L8 (1.5099, -91.5099) -> (-18.4901, -91.5099)
  line L9 (-18.4901, -91.5099) -> (-18.4901, -76.5089)
  arc A1 (-13.489, -71.5099) -> (-18.4901, -76.511) centre (-13.4901, -76.5099) ccw
  dimension "d201" = 10
  dimension "d202" = 5
  dimension "d203" = 5
  constraint concentric A0 A1
  constraint vertical L4
  constraint horizontal L5
  constraint horizontal L6
  constraint vertical L7
  constraint horizontal L8
  constraint vertical L9
  constraint coincident L9 A1.end
  constraint coincident L6 A1.start
  constraint coincident A1 L4.end
  constraint coincident A1 L5.start
  measures "d201" diameter of A1
  measures "d202" distance of A0.centre L4.start
  measures "d203" distance of A0.centre L5.end
extrude "Extrude6'" cut sketch "Sketch15" against normal blind 12 contours A0 S0 S1 L6 L7 L8 L9 | A0 S0 S1 L6 L9 A1 bodies 9 in component "Component"
pattern_circular "C-Pattern4" count 4 over 360 about axis through (45, 45, 75) along (0, 0, -1) of "Extrude6'" in component "Component"
sketch "Sketch16" plane through (0, 0, 80) normal (0, 0, 1) x (-1, 0, 0)
  circle A0 centre (-32, -58) radius 9
  circle A1 centre (-58, -58) radius 9
  line L0 (-52, -11.25) -> (-38, -11.25)
  line L1 (-38, -11.25) -> (-38, -16.25)
  line L2 (-38, -16.25) -> (-52, -16.25)
  line L3 (-52, -16.25) -> (-52, -11.25)
  line L4 (-11.25, -38) -> (-11.25, -52)
  line L5 (-11.25, -52) -> (-16.25, -52)
  line L6 (-16.25, -52) -> (-16.25, -38)
  line L7 (-16.25, -38) -> (-11.25, -38)
  line L8 (-38, -78.75) -> (-52, -78.75)
  line L9 (-52, -78.75) -> (-52, -73.75)
  line L10 (-52, -73.75) -> (-38, -73.75)
  line L11 (-38, -73.75) -> (-38, -78.75)
  line L12 (-78.75, -52) -> (-78.75, -38)
  line L13 (-78.75, -38) -> (-73.75, -38)
  line L14 (-73.75, -38) -> (-73.75, -52)
  line L15 (-73.75, -52) -> (-78.75, -52)
  circle A2 centre (-45, -45) radius 110
sketch "Sketch17" plane through (0, -5, 0) normal (0, -1, 0) x (1, 0, 0)
  arc A0 (90.263, -14.1987) -> (99.6599, -20.7785) centre (99.6599, -10.7785) ccw
  line L0 (99.6599, -20.7785) -> (113.9414, -20.7785)
  line L1 (113.9414, -20.7785) -> (95.643, 29.496)
  arc A1 (95.643, 29.496) -> (81.5476, 39.3657) centre (81.5476, 24.3657) ccw
  line L2 (81.5476, 39.3657) -> (8.4524, 39.3657)
  arc A2 (8.4524, 39.3657) -> (-5.643, 29.496) centre (8.4524, 24.3657) ccw
  line L3 (-5.643, 29.496) -> (-23.9414, -20.7785)
  line L4 (-23.9414, -20.7785) -> (-9.6599, -20.7785)
  arc A3 (-9.6599, -20.7785) -> (-0.263, -14.1987) centre (-9.6599, -10.7785) ccw
  line L5 (-0.263, -14.1987) -> (8.3612, 9.496)
  arc A4 (22.4566, 19.3657) -> (8.3612, 9.496) centre (22.4566, 4.3657) ccw
  line L6 (22.4566, 19.3657) -> (67.5434, 19.3657)
  arc A5 (81.6388, 9.496) -> (67.5434, 19.3657) centre (67.5434, 4.3657) ccw
  line L7 (81.6388, 9.496) -> (90.263, -14.1987)
  line L8 (90, 30) -> (90, 20)
  line L9 (90, 20) -> (85, 20)
  line L10 (85, 20) -> (85, 30)
  line L11 (85, 30) -> (90, 30)
  line L12 (5, 20) -> (0, 20)
  line L13 (0, 20) -> (0, 30)
  line L14 (0, 30) -> (5, 30)
  line L15 (5, 30) -> (5, 20)
sketch "Sketch18" plane through (0, 0, 0) normal (-1, 0, 0) x (0, -1, 0)
  line L0 (-80, 50) -> (-90, 50)
  line L1 (-90, 50) -> (-90, 40)
  line L2 (-90, 40) -> (-85, 40)
  line L3 (-85, 40) -> (-85, 30)
  line L4 (-85, 30) -> (-95, 30)
  line L5 (-95, 30) -> (-95, 20)
  line L6 (-95, 20) -> (-85, 20)
  line L7 (-85, 20) -> (-85, 10)
  line L8 (-85, 10) -> (-90, 10)
  line L9 (-90, 10) -> (-90, 0)
  line L10 (-90, 0) -> (-80, 0)
  line L11 (-80, 0) -> (-80, 5)
  line L12 (-80, 5) -> (-70, 5)
  line L13 (-70, 5) -> (-70, 0)
  line L14 (-70, 0) -> (-60, 0)
  line L15 (-60, 0) -> (-60, 5)
  line L16 (-60, 5) -> (-50, 5)
  line L17 (-50, 5) -> (-50, 0)
  line L18 (-50, 0) -> (-40, 0)
  line L19 (-40, 0) -> (-40, 5)
  line L20 (-40, 5) -> (-35, 5)
  line L21 (-35, 5) -> (-30, 5)
  line L22 (-30, 5) -> (-30, 0)
  line L23 (-30, 0) -> (-20, 0)
  line L24 (-20, 0) -> (-20, 5)
  line L25 (-20, 5) -> (-10, 5)
  line L26 (-10, 5) -> (-10, 0)
  line L27 (-10, 0) -> (-5, 0)
  line L28 (-5, 0) -> (0, 0)
  line L29 (0, 0) -> (0, 10)
  line L30 (0, 10) -> (-5, 10)
  line L31 (-5, 10) -> (-5, 20)
  line L32 (-5, 20) -> (5, 20)
  line L33 (5, 20) -> (5, 30)
  line L34 (5, 30) -> (-5, 30)
  line L35 (-5, 30) -> (-5, 40)
  line L36 (-5, 40) -> (0, 40)
  line L37 (0, 40) -> (0, 50)
  line L38 (0, 50) -> (-5, 50)
  line L39 (-5, 50) -> (-10, 50)
  line L40 (-10, 50) -> (-10, 45)
  line L41 (-10, 45) -> (-20, 45)
  line L42 (-20, 45) -> (-20, 50)
  line L43 (-20, 50) -> (-30, 50)
  line L44 (-30, 50) -> (-30, 45)
  line L45 (-30, 45) -> (-40, 45)
  line L46 (-40, 45) -> (-40, 50)
  line L47 (-40, 50) -> (-50, 50)
  line L48 (-50, 50) -> (-50, 45)
  line L49 (-50, 45) -> (-60, 45)
  line L50 (-60, 45) -> (-60, 50)
  line L51 (-60, 50) -> (-70, 50)
  line L52 (-70, 50) -> (-70, 45)
  line L53 (-70, 45) -> (-80, 45)
  line L54 (-80, 45) -> (-80, 50)
sketch "Sketch19" plane through (0, 0, 0) normal (0, -1, 0) x (1, 0, 0)
  line L0 (60, 5) -> (60, 0)
  line L1 (60, 0) -> (70, 0)
  line L2 (70, 0) -> (70, 5)
  line L3 (70, 5) -> (80, 5)
  line L4 (80, 5) -> (80, 0)
  line L5 (80, 0) -> (85, 0)
  line L6 (85, 0) -> (85, 10)
  line L7 (85, 10) -> (90, 10)
  line L8 (90, 10) -> (90, 20)
  line L9 (90, 20) -> (85, 20)
  line L10 (85, 20) -> (85, 30)
  line L11 (85, 30) -> (90, 30)
  line L12 (90, 30) -> (90, 40)
  line L13 (90, 40) -> (85, 40)
  line L14 (85, 40) -> (85, 50)
  line L15 (85, 50) -> (80, 50)
  line L16 (80, 50) -> (80, 45)
  line L17 (80, 45) -> (70, 45)
  line L18 (70, 45) -> (70, 50)
  line L19 (70, 50) -> (60, 50)
  line L20 (60, 50) -> (60, 45)
  line L21 (60, 45) -> (50, 45)
  line L22 (50, 45) -> (50, 50)
  line L23 (50, 50) -> (40, 50)
  line L24 (40, 50) -> (40, 45)
  line L25 (40, 45) -> (30, 45)
  line L26 (30, 45) -> (30, 50)
  line L27 (30, 50) -> (20, 50)
  line L28 (20, 50) -> (20, 45)
  line L29 (20, 45) -> (10, 45)
  line L30 (10, 45) -> (10, 50)
  line L31 (10, 50) -> (5, 50)
  line L32 (5, 50) -> (5, 40)
  line L33 (5, 40) -> (0, 40)
  line L34 (0, 40) -> (0, 30)
  line L35 (0, 30) -> (5, 30)
  line L36 (5, 30) -> (5, 20)
  line L37 (5, 20) -> (0, 20)
  line L38 (0, 20) -> (0, 10)
  line L39 (0, 10) -> (5, 10)
  line L40 (5, 10) -> (5, 0)
  line L41 (5, 0) -> (10, 0)
  line L42 (10, 0) -> (10, 5)
  line L43 (10, 5) -> (20, 5)
  line L44 (20, 5) -> (20, 0)
  line L45 (20, 0) -> (30, 0)
  line L46 (30, 0) -> (30, 5)
  line L47 (30, 5) -> (40, 5)
  line L48 (40, 5) -> (40, 0)
  line L49 (40, 0) -> (50, 0)
  line L50 (50, 0) -> (50, 5)
  line L51 (50, 5) -> (60, 5)